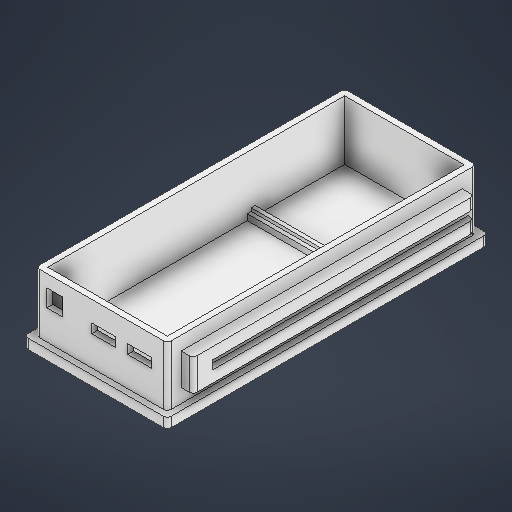
# Autodesk Inventor part: module_switch
Saved by Autodesk Inventor 2025.2 (Build 292293000, 293)
## iProperties
Created: 2025-09-07
Part Number: module_switch
Material: PC/ABS Plastic
Document SubType Name: Modeling
Designer: sam
Density: 1.1 g/cm^3
Appearance: Smooth - White
Author: sam
Autodesk Inventor part; units mm, degrees
ref_plane "YZ Plane" through (0, 0, 0) normal (1, 0, 0) x (0, 1, 0)
ref_plane "XZ Plane" through (0, 0, 0) normal (0, 1, 0) x (-1, 0, 0)
ref_plane "XY Plane" through (0, 0, 0) normal (0, 0, 1) x (1, 0, 0)
sketch "Sketch2" plane through (0, 0, 0) normal (0, 1, 0) x (-1, 0, 0)
  line L0 (-36.2, -81) -> (36.2, -81)
  line L1 (36.2, -81) -> (36.2, 81)
  line L2 (36.2, 81) -> (-36.2, 81)
  line L3 (-36.2, 81) -> (-36.2, -81)
  line L4 (-36.2, -81) -> (36.2, 81) construction
  line L5 (36.2, -81) -> (-36.2, 81) construction
  point P0 (0, 0)
  dimension "d0" = 72.4
  dimension "d1" = 162
  constraints: 12 end point, 2 midpoint, 2 parallel, 1 horizontal, 1 perpendicular
  measures "d0" distance of L2.end L1.end
  measures "d1" distance of L1.end L0.end
extrude "Extrusion1" add sketch "Sketch2" along normal blind 5
sketch "Sketch3" plane through (0, 5, 0) normal (0, 1, 0) x (1, 0, 0)
  line L0 (33.2, 78) -> (-33.2, 78)
  line L1 (-33.2, 78) -> (-33.2, -78)
  line L2 (-33.2, -78) -> (33.2, -78)
  line L3 (33.2, -78) -> (33.2, 78)
  line L4 (33.2, 78) -> (-33.2, -78) construction
  line L5 (-33.2, 78) -> (33.2, -78) construction
  line L6 (-36.2, 81) -> (-36.2, -81) projected
  line L7 (-36.2, -81) -> (36.2, -81) projected
  line L8 (30.2, 75) -> (-30.2, 75)
  line L9 (-30.2, 75) -> (-30.2, -75)
  line L10 (-30.2, -75) -> (30.2, -75)
  line L11 (30.2, -75) -> (30.2, 75)
  line L12 (30.2, 75) -> (-30.2, -75) construction
  line L13 (-30.2, 75) -> (30.2, -75) construction
  point P0 (0, 0)
  dimension "d4" = 3
  dimension "d5" = 3
  dimension "d6" = 3
  dimension "d7" = 3
  constraints: 24 end point, 4 midpoint, 4 parallel, 2 horizontal, 2 perpendicular
  measures "d4" distance between parallel lines of L6 L1
  measures "d5" distance between parallel lines of L7 L2
  measures "d6" distance between parallel lines of L2 L10
  measures "d7" distance between parallel lines of L1 L9
extrude "Extrusion2" add sketch "Sketch3" along normal blind 30
fillet "Fillet1" radius 2 8 edges at (33.2, 20, 78) (-33.2, 20, 78) (-36.2, 2.5, 81) (36.2, 2.5, 81) (33.2, 20, -78) (-33.2, 20, -78) (36.2, 2.5, -81) (-36.2, 2.5, -81)
sketch "Sketch4" plane through (33.2, 5, 76) normal (1, 0, 0) x (0, 0, -1)
  line L0 (5, 23) -> (147, 23)
  line L1 (147, 23) -> (147, 7)
  line L2 (147, 7) -> (5, 7)
  line L3 (5, 7) -> (5, 23)
  line L4 (152, 30) -> (152, 0) projected
  line L5 (0, 30) -> (152, 30) projected
  line L6 (0, 0) -> (0, 30) projected
  line L7 (152, 0) -> (0, 0) projected
  line L8 (-5, 0) -> (-5, -5) projected
  line L9 (157, -5) -> (157, 0) projected
  point P0 (76, -5)
  point P1 (0, 15)
  dimension "d42" = 10
  dimension "d43" = 10
  dimension "d44" = 16
  dimension "d45" = 8
  constraints: 8 end point, 2 parallel, 1 horizontal, 1 midpoint, 1 perpendicular
  measures "d42" distance between parallel lines of L8 L3
  measures "d43" distance between parallel lines of L9 L1
  measures "d44" distance between parallel lines of L0 L2
  measures "d45" distance from line of point (0, 15) L0
extrude "Extrusion3" add sketch "Sketch4" along normal blind 6 contours L0 L1 L2 L3
sketch "Sketch5" plane through (33.2, 12, -71) normal (0, 0, -1) x (-1, 0, 0)
  line L0 (0, 16) -> (0, 0) projected
  line L1 (0, 16) -> (-6, 16) projected
  line L2 (-6, 0) -> (-6, 16) projected
  line L3 (0, 0) -> (-6, 0) projected
  line L4 (-6, 16) -> (0, 16)
  line L5 (0, 16) -> (0, 13.2)
  line L6 (0, 13.2) -> (-6, 13.2)
  line L7 (-6, 13.2) -> (-6, 16)
  line L8 (-6, 0) -> (0, 0)
  line L9 (0, 0) -> (0, 2.8)
  line L10 (0, 2.8) -> (-6, 2.8)
  line L11 (-6, 2.8) -> (-6, 0)
  line L12 (-6, 2.8) -> (-3, 2.8)
  line L13 (-3, 2.8) -> (-3, 5.8)
  line L14 (-3, 5.8) -> (-6, 5.8)
  line L15 (-6, 5.8) -> (-6, 2.8)
  line L16 (-6, 13.2) -> (-3, 13.2)
  line L17 (-3, 13.2) -> (-3, 10.2)
  line L18 (-3, 10.2) -> (-6, 10.2)
  line L19 (-6, 10.2) -> (-6, 13.2)
  point P0 (33.2, -12)
  point P1 (0, 11)
  dimension "d99" = 2.8
  dimension "d100" = 2.8
  dimension "d101" = 3
  dimension "d102" = 3
  dimension "d103" = 3
  dimension "d104" = 3
  constraints: 32 end point, 8 parallel, 4 horizontal, 4 perpendicular, 3 point on line
  measures "d99" distance of L4.end L5.end
  measures "d100" distance of L9.end L8.end
  measures "d101" distance of L14.end L13.end
  measures "d102" distance of L13.end L12.end
  measures "d103" distance of L17.end L18.end
  measures "d104" distance of L16.end L17.end
extrude "Extrusion4" cut sketch "Sketch5" against normal blind 132 contours L0 L10 L13 L14 L2 L18 L17 L6
sketch "Sketch6" plane through (-33.2, 5, -76) normal (-1, 0, 0) x (0, 0, 1)
  line L0 (0, 0) -> (0, 30) projected
  line L1 (152, 0) -> (0, 0) projected
  line L2 (152, 30) -> (152, 0) projected
  line L3 (0, 30) -> (152, 30) projected
  line L4 (5, 20) -> (137, 20)
  line L5 (137, 20) -> (137, 10)
  line L6 (137, 10) -> (5, 10)
  line L7 (5, 10) -> (5, 20)
  line L8 (157, -5) -> (157, 0) projected
  line L9 (-5, 0) -> (-5, -5) projected
  point P0 (76, -5)
  point P1 (0, 15)
  dimension "d48" = 20
  dimension "d49" = 10
  dimension "d50" = 5
  dimension "d51" = 10
  constraints: 8 end point, 2 parallel, 1 horizontal, 1 midpoint, 1 perpendicular
  measures "d48" distance between parallel lines of L8 L5
  measures "d49" distance between parallel lines of L9 L7
  measures "d50" distance from line of point (0, 15) L4
  measures "d51" distance between parallel lines of L6 L4
extrude "Extrusion5" add sketch "Sketch6" along normal blind 6 contours L4 L5 L6 L7
sketch "Sketch7" plane through (-33.2, 15, 61) normal (0, 0, 1) x (1, 0, 0)
  line L0 (0, 10) -> (0, 0) projected
  line L1 (0, 10) -> (-6, 10) projected
  line L2 (-6, 0) -> (-6, 10) projected
  line L3 (0, 0) -> (-6, 0) projected
  line L4 (0, 10) -> (-3.4, 10)
  line L5 (-3.4, 10) -> (-3.4, 7)
  line L6 (-3.4, 7) -> (0, 7)
  line L7 (0, 7) -> (0, 10)
  line L8 (0, 0) -> (-3.4, 0)
  line L9 (-3.4, 0) -> (-3.4, 3)
  line L10 (-3.4, 3) -> (0, 3)
  line L11 (0, 3) -> (0, 0)
  point P0 (33.2, -15)
  point P1 (-3.4, 0)
  point P2 (0, 7)
  dimension "d30" = 3.4
  dimension "d31" = 3
  dimension "d32" = 3.4
  dimension "d33" = 3
  constraints: 16 end point, 4 parallel, 2 horizontal, 2 perpendicular
  measures "d30" distance of L6.end L5.end
  measures "d31" distance of L5.end L4.end
  measures "d32" distance of L9.end L10.end
  measures "d33" distance of L8.end L9.end
extrude "Extrusion6" cut sketch "Sketch7" against normal up to surface (132 mm away) contours L0 L6 L5 L1 | L0 L3 L9 L10
fillet "Fillet3" radius 1 4 edges at (-34.9, 22, -71) (-34.9, 18, -71) (-34.9, 22, 61) (-34.9, 18, 61)
fillet "Fillet4" radius 1 4 edges at (-39.2, 25, -5) (-36.6, 25, -5) (-39.2, 15, -5) (-36.6, 15, -5)
fillet "Fillet5" radius 2 3 edges at (39.2, 20, 71) (39.2, 25.1, -71) (39.2, 14.9, -71)
fillet "Fillet6" radius 1 11 edges at (-38.9071, 24.7071, 61) (-37.9, 25, 61) (-36.8929, 24.7071, 61) (-36.6, 21.5, 61) (-36.6, 23, 61) (-38.9071, 15.2929, 61) (-37.9, 15, 61) (-36.8929, 15.2929, 61) (-36.6, 17, 61) (-36.6, 18.5, 61) (-39.2, 20, 61)
fillet "Fillet7" radius 1 11 edges at (-36.8929, 24.7071, -71) (-37.9, 25, -71) (-38.9071, 24.7071, -71) (-39.2, 20, -71) (-38.9071, 15.2929, -71) (-37.9, 15, -71) (-36.8929, 15.2929, -71) (-36.6, 18.5, -71) (-36.6, 17, -71) (-36.6, 23, -71) (-36.6, 21.5, -71)
sketch "Sketch10" plane through (0, 5, 0) normal (0, 1, 0) x (1, 0, 0)
  line L0 (30.2, 75) -> (-30.2, 75) projected
  line L1 (-30.2, 75) -> (-30.2, -75) projected
  line L2 (-30.2, -75) -> (30.2, -75) projected
  line L3 (30.2, -75) -> (30.2, 75) projected
  line L4 (-30.2, -75) -> (30.2, -75)
  line L5 (30.2, -75) -> (30.2, -70.6)
  line L6 (30.2, -70.6) -> (-30.2, -70.6)
  line L7 (-30.2, -70.6) -> (-30.2, -75)
  line L8 (-30.2, -70.6) -> (30.2, -70.6)
  line L9 (30.2, -70.6) -> (30.2, 25.8)
  line L10 (30.2, 25.8) -> (-30.2, 25.8)
  line L11 (-30.2, 25.8) -> (-30.2, -70.6)
  line L12 (-30.2, 25.8) -> (30.2, 25.8)
  line L13 (30.2, 25.8) -> (30.2, 29.8)
  line L14 (30.2, 29.8) -> (-30.2, 29.8)
  line L15 (-30.2, 29.8) -> (-30.2, 25.8)
  point P0 (0, 0)
  point P1 (-30.2, 29.8)
  point P2 (-30.2, 25.8)
  dimension "d90" = 4.4
  dimension "d91" = 96.4
  dimension "d92" = 4
  constraints: 24 end point, 6 parallel, 3 horizontal, 3 perpendicular, 3 point on line
  measures "d90" distance of L5.end L4.end
  measures "d91" distance of L9.end L8.end
  measures "d92" distance of L13.end L12.end
extrude "Extrusion9" add sketch "Sketch10" along normal blind 3 contours L3 L10 L1 L14 | L3 L2 L1 L6
sketch "Sketch11" plane through (0, 8, 0) normal (0, 1, 0) x (1, 0, 0)
  line L0 (-30.2, 25.8) -> (-30.2, 29.8) projected
  line L1 (-30.2, 25.8) -> (30.2, 25.8) projected
  line L2 (30.2, 29.8) -> (30.2, 25.8) projected
  line L3 (30.2, 29.8) -> (-30.2, 29.8) projected
  line L4 (-30.2, -75) -> (-30.2, -70.6) projected
  line L5 (30.2, -75) -> (-30.2, -75) projected
  line L6 (30.2, -70.6) -> (30.2, -75) projected
  line L7 (30.2, -70.6) -> (-30.2, -70.6) projected
  line L8 (30.2, 29.8) -> (-30.2, 29.8) projected
  line L9 (-30.2, 29.8) -> (30.2, 29.8)
  line L10 (30.2, 29.8) -> (30.2, 27.8)
  line L11 (30.2, 27.8) -> (-30.2, 27.8)
  line L12 (-30.2, 27.8) -> (-30.2, 29.8)
  line L13 (-30.2, -75) -> (30.2, -75)
  line L14 (30.2, -75) -> (30.2, -72.6)
  line L15 (30.2, -72.6) -> (-30.2, -72.6)
  line L16 (-30.2, -72.6) -> (-30.2, -75)
  point P0 (0, 0)
  dimension "d95" = 2
  dimension "d96" = 2.4
  constraints: 16 end point, 4 parallel, 2 horizontal, 2 perpendicular, 1 midpoint, 1 point on line
  measures "d95" distance of L9.end L10.end
  measures "d96" distance of L14.end L13.end
extrude "Extrusion10" add sketch "Sketch11" along normal blind 1.6 contours L0 L3 L2 L11 | L4 L15 L6 L5
sketch "Sketch12" plane through (-31.2, 5, 78) normal (0, 0, 1) x (1, 0, 0)
  line L0 (-2, 30) -> (-2, 0) projected
  line L1 (0, 30) -> (62.4, 30) projected
  line L2 (-2, 30) -> (0, 30) projected
  line L3 (62.4, 30) -> (64.4, 30) projected
  line L4 (64.4, 0) -> (64.4, 30) projected
  line L5 (62.4, 0) -> (0, 0) projected
  line L6 (0, 0) -> (-2, 0) projected
  line L7 (64.4, 0) -> (62.4, 0) projected
  line L8 (56.4, 19.7) -> (44.3, 19.7)
  line L9 (44.3, 19.7) -> (44.3, 15)
  line L10 (44.3, 15) -> (56.4, 15)
  line L11 (56.4, 15) -> (56.4, 19.7)
  line L12 (38.3, 19.7) -> (26.2, 19.7)
  line L13 (26.2, 19.7) -> (26.2, 15)
  line L14 (26.2, 15) -> (38.3, 15)
  line L15 (38.3, 15) -> (38.3, 19.7)
  line L16 (3.5, 23.7) -> (11.56, 23.7)
  line L17 (11.56, 23.7) -> (11.56, 15)
  line L18 (11.56, 15) -> (3.5, 15)
  line L19 (3.5, 15) -> (3.5, 23.7)
  point P0 (31.2, -5)
  dimension "d105" = 12.1
  dimension "d106" = 4.7
  dimension "d107" = 15
  dimension "d108" = 8
  dimension "d109" = 12.1
  dimension "d110" = 4.7
  dimension "d112" = 15
  dimension "d113" = 6
  dimension "d116" = 8.06
  dimension "d117" = 8.7
  dimension "d118" = 15
  dimension "d119" = 5.5
  constraints: 24 end point, 6 parallel, 3 horizontal, 3 perpendicular
  measures "d105" distance of L10.end L9.end
  measures "d106" distance of L9.end L8.end
  measures "d107" distance between parallel lines of L5 L10
  measures "d108" distance between parallel lines of L4 L11
  measures "d109" distance of L14.end L13.end
  measures "d110" distance of L13.end L12.end
  measures "d112" distance between parallel lines of L5 L14
  measures "d113" distance between parallel lines of L9 L15
  measures "d116" distance of L17.end L18.end
  measures "d117" distance of L16.end L17.end
  measures "d118" distance between parallel lines of L5 L18
  measures "d119" distance between parallel lines of L0 L19
extrude "Extrusion11" cut sketch "Sketch12" against normal blind 3 contours L11 L10 L9 L8 | L15 L14 L13 L12 | L16 L17 L18 L19
body "Solid1"
